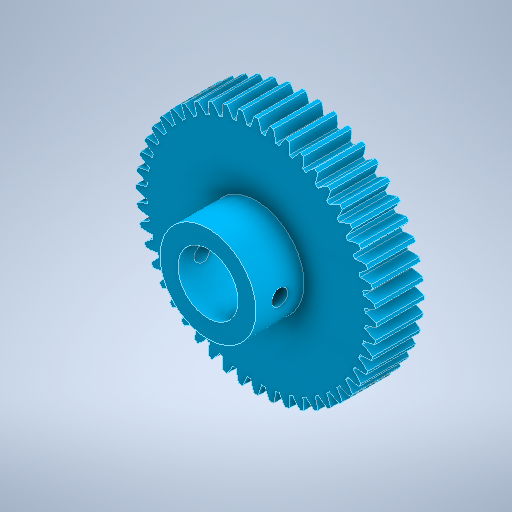
# Autodesk Inventor part: 平歯車2
Saved by Autodesk Inventor 2025.1 (Build 291241000, 241)
## iProperties
CustomPartVersion: 1
Created: 2024-10-03
Part Number: 平歯車2
Material: Steel
Document SubType Name: Modeling
Designer: yuki0520
Categories: <?xml version="1.0" encoding="UTF-16"?> <MemberInstance><Categories><FamilyTemplate><FamilyTemplateParameter ValueType="xs:double" Id="1" ObjectReferenceKey="da_z" ObjectType="kUserParameterObject"/><FamilyTemplateParameter ValueType="xs:double" Id="2" ObjectReferenceKey="da_b" ObjectType="kUserParameterObject"/><FamilyTemplateParameter ValueType="xs:double" Id="3" ObjectReferenceKey="da_beta" ObjectType="kUserParameterObject"/><FamilyTemplateParameter ValueType="xs:double" Id="4" ObjectReferenceKey="da_da" ObjectType="kUserParameterObject"/><FamilyTemplateParameter ValueType="xs:double" Id="5" ObjectReferenceKey="da_aw" ObjectType="kUserParameterObject"/><FamilyTemplateParameter ValueType="xs:string" Id="6" ObjectReferenceKey="EAIAABAAAACIAQAAAAAAAIAAAAAAAAAA" ObjectType="83910656" SubObjectId="SurfaceGeometry"/></FamilyTemplate><ParamToTemplateMap><ParamToTemplate CategoryParameter="//CategoryParameter[@InternalName='046C89C9-8512-4d59-83FE-43B91F4F132A']" TemplateParameter="1"/><ParamToTemplate CategoryParameter="//CategoryParameter[@InternalName='2552DF32-E462-4b46-AEBF-C6C7768E72AC']" TemplateParameter="2"/><ParamToTemplate CategoryParameter="//CategoryParameter[@InternalName='C9EE641D-15FC-4fae-A226-E94C4372FDD7']" TemplateParameter="3"/><ParamToTemplate><ParamToTemplate CategoryParameter="//CategoryParameter[@InternalName='00B6519A-459B-49c7-AD84-2E56D39A5744']" ConstantValue="0.000000"/></ParamToTemplate><ParamToTemplate><ParamToTemplate CategoryParameter="//CategoryParameter[@InternalName='04B31F0E-C7A6-4894-AA32-9629BEFACF47']" ConstantValue="1.000000"/></ParamToTemplate><ParamToTemplate><ParamToTemplate CategoryParameter="//CategoryParameter[@InternalName='43CBEC2E-7847-49e7-A936-2F7889FCB2D9']" ConstantValue="0.250000"/></ParamToTemplate><ParamToTemplate><ParamToTemplate CategoryParameter="//CategoryParameter[@InternalName='B1EFC894-105D-4ebd-86BF-FA20ED196853']" ConstantValue="0.350000"/></ParamToTemplate><ParamToTemplate><ParamToTemplate CategoryParameter="//CategoryParameter[@InternalName='51175063-3D10-4879-93E8-6246FE8B403D']" ConstantValue="2060000000.000000"/></ParamToTemplate><ParamToTemplate><ParamToTemplate CategoryParameter="//CategoryParameter[@InternalName='A3A52E27-4454-46a9-B0BD-C932399B70AF']" ConstantValue="0.300000"/></ParamToTemplate><ParamToTemplate><ParamToTemplate CategoryParameter="//CategoryParameter[@InternalName='91B76062-C214-41d9-B1B9-14D2AB99603D']" ConstantValue="0.100000"/></ParamToTemplate><ParamToTemplate><ParamToTemplate CategoryParameter="//CategoryParameter[@InternalName='374E806E-8B8A-4dda-A9AA-1039D6500AD2']" ConstantValue="10.000000"/></ParamToTemplate><ParamToTemplate><ParamToTemplate CategoryParameter="//CategoryParameter[@InternalName='2D373A89-B862-43d6-8D0B-0CBF12AB9F6C']" ConstantValue="0.349066"/></ParamToTemplate><ParamToTemplate CategoryParameter="//CategoryParameter[@InternalName='37777632-D6A2-4fac-9D53-DB8ACD95C989']" TemplateParameter="4"/><ParamToTemplate CategoryParameter="//CategoryParameter[@InternalName='FD1017F1-B727-4f7e-9707-0F86F1FF9423']" TemplateParameter="5"/><ParamToTemplate><ParamToTemplate CategoryParameter="//CategoryParameter[@InternalName='9E1B4470-B2D3-4ff1-B813-535BB4CDF51A']" ConstantValue="3520000.000000"/></ParamToTemplate><ParamToTemplate><ParamToTemplate CategoryParameter="//CategoryParameter[@InternalName='F8452263-BFF6-458c-9FB1-07C4B99E95CD']" ConstantValue="11400000.000000"/></ParamToTemplate><ParamToTemplate><ParamToTemplate CategoryParameter="//CategoryParameter[@InternalName='3E3BB259-FD49-497f-8171-6EBC954A3479']" ConstantValue="2.000000"/></ParamToTemplate><ParamToTemplate CategoryParameter="//CategoryParameter[@InternalName='27C3BAF2-7550-4e4b-AE2C-0DB134B7D9B7']" TemplateParameter="6"/></ParamToTemplateMap><Category DisplayName="Gear" InternalName="DC85795E-93AB-48d5-8EEE-5A27447B64BD" Mnemonic="Gear"><CategoryParameter DisplayName="z" InternalName="046C89C9-8512-4d59-83FE-43B91F4F132A" Mnemonic="z"/><CategoryParameter DisplayName="b" InternalName="2552DF32-E462-4b46-AEBF-C6C7768E72AC" Mnemonic="b"/><CategoryParameter DisplayName="||b|" InternalName="C9EE641D-15FC-4fae-A226-E94C4372FDD7" Mnemonic="beta"/><CategoryParameter DisplayName="x" InternalName="00B6519A-459B-49c7-AD84-2E56D39A5744" Mnemonic="x"/><CategoryParameter DisplayName="a*" InternalName="04B31F0E-C7A6-4894-AA32-9629BEFACF47" Mnemonic="a"/><CategoryParameter DisplayName="c*" InternalName="43CBEC2E-7847-49e7-A936-2F7889FCB2D9" Mnemonic="c"/><CategoryParameter DisplayName="r|.f|*" InternalName="B1EFC894-105D-4ebd-86BF-FA20ED196853" Mnemonic="rf"/><CategoryParameter DisplayName="E" InternalName="51175063-3D10-4879-93E8-6246FE8B403D" Mnemonic="E"/><CategoryParameter DisplayName="||m|" InternalName="A3A52E27-4454-46a9-B0BD-C932399B70AF" Mnemonic="mi"/><Category DisplayName="SpurGear" InternalName="26C5A22E-A91E-4dfd-A3B3-23CCAFAE1764" Mnemonic="SpurGear"><CategoryParameter DisplayName="m" InternalName="91B76062-C214-41d9-B1B9-14D2AB99603D" Mnemonic="m"/><CategoryParameter DisplayName="P" InternalName="374E806E-8B8A-4dda-A9AA-1039D6500AD2" Mnemonic="PP"/><CategoryParameter DisplayName="||a|" InternalName="2D373A89-B862-43d6-8D0B-0CBF12AB9F6C" Mnemonic="alpha"/><CategoryParameter DisplayName="d|.a|" InternalName="37777632-D6A2-4fac-9D53-DB8ACD95C989" Mnemonic="da"/><CategoryParameter DisplayName="a|.w|" InternalName="FD1017F1-B727-4f7e-9707-0F86F1FF9423" Mnemonic="aw"/><CategoryParameter DisplayName="||s||.Flim|" InternalName="9E1B4470-B2D3-4ff1-B813-535BB4CDF51A" Mnemonic="sFlim"/><CategoryParameter DisplayName="||s||.Hlim|" InternalName="F8452263-BFF6-458c-9FB1-07C4B99E95CD" Mnemonic="sHlim"/><CategoryParameter DisplayName="タイプ" InternalName="3E3BB259-FD49-497f-8171-6EBC954A3479" Mnemonic="type"/><CategoryParameter DisplayName="PitchDiameter" InternalName="27C3BAF2-7550-4e4b-AE2C-0DB134B7D9B7" Mnemonic="IDS_PITCHDIAM"/></Category></Category></Categories></MemberInstance>
Density: 1 g/cm^3
Appearance: スカイ ブルー 標準
Author: yuki0520
Autodesk Inventor part; units mm, degrees
sketch "Sketch1" plane through (0, 0, 0) normal (0, 0, 1) x (1, 0, 0)
  circle A0 centre (0, 0) radius 25
  dimension "d0" = 50
  constraints: 1 centre point
  measures "d0" diameter of A0
extrude "Extrusion1" add sketch "Sketch1" along normal blind 10
ref_plane "Work Plane2" through (0, 0, 5) normal (0, 0, 1) x (1, 0, 0)
sketch "Sketch2" plane through (0, 0, 0) normal (0, 0, -1) x (-1, 0, 0)
  circle A0 centre (0, 0) radius 25 projected
  circle A1 centre (0, 0) radius 24
  dimension "d3" = 48
  constraints: 1 centre point, 1 coincident
  measures "d3" diameter of A1
surface extrude "ピッチ円直径" sketch "Sketch2" against normal through all shown no curves A1
ref_plane "Work Plane8" through (0, 0, 0) normal (0.9978589, 0.0654031, 0) x (0, 0, 1)
ref_plane "Work Plane9" through (0, 0, 0) normal (1, 0, 0) x (0, 1, 0)
spur gear teeth "平歯車" teeth 48 pitch diameter 48 tip diameter 50 root diameter 45.5 face width 10 start plane through (0, 0, 0) normal (0, 0, -1) x (-1, 0, 0)
sketch "スケッチ3" plane through (0, 0, 10) normal (0, 0, 1) x (1, 0, 0)
  circle A0 centre (0, 0) radius 6
  circle A1 centre (0, 0) radius 10
  arc A2 (3.6683, -24.7294) -> (4.0726, -22.3825) centre (-7.7435, -21.5549) ccw projected
  arc A3 (4.0726, -22.3825) -> (4.8028, -22.2373) centre (0, 0) ccw projected
  arc A4 (4.8028, -22.2373) -> (6.0745, -24.2508) centre (15.4028, -16.9508) ccw projected
  arc A5 (6.0745, -24.2508) -> (6.8647, -24.039) centre (0, 0) ccw projected
  arc A6 (6.8647, -24.039) -> (6.9593, -21.6594) centre (-4.8638, -22.3812) ccw projected
  arc A7 (6.9593, -21.6594) -> (7.6642, -21.4201) centre (0, 0) ccw projected
  arc A8 (7.6642, -21.4201) -> (9.1879, -23.2504) centre (17.4835, -14.7953) ccw projected
  arc A9 (9.1879, -23.2504) -> (9.9437, -22.9374) centre (0, 0) ccw projected
  arc A10 (9.9437, -22.9374) -> (9.7269, -20.5658) centre (-1.9009, -22.8246) ccw projected
  arc A11 (9.7269, -20.5658) -> (10.3946, -20.2365) centre (0, 0) ccw projected
  arc A12 (10.3946, -20.2365) -> (12.1441, -21.8523) centre (19.2651, -12.3867) ccw projected
  arc A13 (12.1441, -21.8523) -> (12.8526, -21.4432) centre (0, 0) ccw projected
  arc A14 (12.8526, -21.4432) -> (12.328, -19.1202) centre (1.0946, -22.8774) ccw projected
  arc A15 (12.328, -19.1202) -> (12.947, -18.7066) centre (0, 0) ccw projected
  arc A16 (12.947, -18.7066) -> (14.8925, -20.0802) centre (20.7171, -9.7661) ccw projected
  arc A17 (14.8925, -20.0802) -> (15.5415, -19.5822) centre (0, 0) ccw projected
  arc A18 (15.5415, -19.5822) -> (14.7183, -17.3475) centre (4.0714, -22.5388) ccw projected
  arc A19 (14.7183, -17.3475) -> (15.278, -16.8566) centre (0, 0) ccw projected
  arc A20 (15.278, -16.8566) -> (17.3861, -17.9645) centre (21.8146, -6.9784) ccw projected
  arc A21 (17.3861, -17.9645) -> (17.9645, -17.3861) centre (0, 0) ccw projected
  arc A22 (17.9645, -17.3861) -> (16.8566, -15.278) centre (6.9784, -21.8146) ccw projected
  arc A23 (16.8566, -15.278) -> (17.3475, -14.7183) centre (0, 0) ccw projected
  arc A24 (17.3475, -14.7183) -> (19.5822, -15.5415) centre (22.5388, -4.0714) ccw projected
  arc A25 (19.5822, -15.5415) -> (20.0802, -14.8925) centre (0, 0) ccw projected
  arc A26 (20.0802, -14.8925) -> (18.7066, -12.947) centre (9.7661, -20.7171) ccw projected
  arc A27 (18.7066, -12.947) -> (19.1202, -12.328) centre (0, 0) ccw projected
  arc A28 (19.1202, -12.328) -> (21.4432, -12.8526) centre (22.8774, -1.0946) ccw projected
  arc A29 (21.4432, -12.8526) -> (21.8523, -12.1441) centre (0, 0) ccw projected
  arc A30 (21.8523, -12.1441) -> (20.2365, -10.3946) centre (12.3867, -19.2651) ccw projected
  arc A31 (20.2365, -10.3946) -> (20.5658, -9.7269) centre (0, 0) ccw projected
  arc A32 (20.5658, -9.7269) -> (22.9374, -9.9437) centre (22.8246, 1.9009) ccw projected
  arc A33 (22.9374, -9.9437) -> (23.2504, -9.1879) centre (0, 0) ccw projected
  arc A34 (23.2504, -9.1879) -> (21.4201, -7.6642) centre (14.7953, -17.4835) ccw projected
  arc A35 (21.4201, -7.6642) -> (21.6594, -6.9593) centre (0, 0) ccw projected
  arc A36 (21.6594, -6.9593) -> (24.039, -6.8647) centre (22.3812, 4.8638) ccw projected
  arc A37 (24.039, -6.8647) -> (24.2508, -6.0745) centre (0, 0) ccw projected
  arc A38 (24.2508, -6.0745) -> (22.2373, -4.8028) centre (16.9508, -15.4028) ccw projected
  arc A39 (22.2373, -4.8028) -> (22.3825, -4.0726) centre (0, 0) ccw projected
  arc A40 (22.3825, -4.0726) -> (24.7294, -3.6683) centre (21.5549, 7.7435) ccw projected
  arc A41 (24.7294, -3.6683) -> (24.8362, -2.8572) centre (0, 0) ccw projected
  arc A42 (24.8362, -2.8572) -> (22.6739, -1.8592) centre (18.8162, -13.0585) ccw projected
  arc A43 (22.6739, -1.8592) -> (22.7226, -1.1163) centre (0, 0) ccw projected
  arc A44 (22.7226, -1.1163) -> (24.9967, -0.409) centre (20.3597, 10.4907) ccw projected
  arc A45 (24.9967, -0.409) -> (24.9967, 0.409) centre (0, 0) ccw projected
  arc A46 (24.9967, 0.409) -> (22.7226, 1.1163) centre (20.3597, -10.4907) ccw projected
  arc A47 (22.7226, 1.1163) -> (22.6739, 1.8592) centre (0, 0) ccw projected
  arc A48 (22.6739, 1.8592) -> (24.8362, 2.8572) centre (18.8162, 13.0585) ccw projected
  arc A49 (24.8362, 2.8572) -> (24.7294, 3.6683) centre (0, 0) ccw projected
  arc A50 (24.7294, 3.6683) -> (22.3825, 4.0726) centre (21.5549, -7.7435) ccw projected
  arc A51 (22.3825, 4.0726) -> (22.2373, 4.8028) centre (0, 0) ccw projected
  arc A52 (22.2373, 4.8028) -> (24.2508, 6.0745) centre (16.9508, 15.4028) ccw projected
  arc A53 (24.2508, 6.0745) -> (24.039, 6.8647) centre (0, 0) ccw projected
  arc A54 (24.039, 6.8647) -> (21.6594, 6.9593) centre (22.3812, -4.8638) ccw projected
  arc A55 (21.6594, 6.9593) -> (21.4201, 7.6642) centre (0, 0) ccw projected
  arc A56 (21.4201, 7.6642) -> (23.2504, 9.1879) centre (14.7953, 17.4835) ccw projected
  arc A57 (23.2504, 9.1879) -> (22.9374, 9.9437) centre (0, 0) ccw projected
  arc A58 (22.9374, 9.9437) -> (20.5658, 9.7269) centre (22.8246, -1.9009) ccw projected
  arc A59 (20.5658, 9.7269) -> (20.2365, 10.3946) centre (0, 0) ccw projected
  arc A60 (20.2365, 10.3946) -> (21.8523, 12.1441) centre (12.3867, 19.2651) ccw projected
  arc A61 (21.8523, 12.1441) -> (21.4432, 12.8526) centre (0, 0) ccw projected
  arc A62 (21.4432, 12.8526) -> (19.1202, 12.328) centre (22.8774, 1.0946) ccw projected
  arc A63 (19.1202, 12.328) -> (18.7066, 12.947) centre (0, 0) ccw projected
  arc A64 (18.7066, 12.947) -> (20.0802, 14.8925) centre (9.7661, 20.7171) ccw projected
  arc A65 (20.0802, 14.8925) -> (19.5822, 15.5415) centre (0, 0) ccw projected
  arc A66 (19.5822, 15.5415) -> (17.3475, 14.7183) centre (22.5388, 4.0714) ccw projected
  arc A67 (17.3475, 14.7183) -> (16.8566, 15.278) centre (0, 0) ccw projected
  arc A68 (16.8566, 15.278) -> (17.9645, 17.3861) centre (6.9784, 21.8146) ccw projected
  arc A69 (17.9645, 17.3861) -> (17.3861, 17.9645) centre (0, 0) ccw projected
  arc A70 (17.3861, 17.9645) -> (15.278, 16.8566) centre (21.8146, 6.9784) ccw projected
  arc A71 (15.278, 16.8566) -> (14.7183, 17.3475) centre (0, 0) ccw projected
  arc A72 (14.7183, 17.3475) -> (15.5415, 19.5822) centre (4.0714, 22.5388) ccw projected
  arc A73 (15.5415, 19.5822) -> (14.8925, 20.0802) centre (0, 0) ccw projected
  arc A74 (14.8925, 20.0802) -> (12.947, 18.7066) centre (20.7171, 9.7661) ccw projected
  arc A75 (12.947, 18.7066) -> (12.328, 19.1202) centre (0, 0) ccw projected
  arc A76 (12.328, 19.1202) -> (12.8526, 21.4432) centre (1.0946, 22.8774) ccw projected
  arc A77 (12.8526, 21.4432) -> (12.1441, 21.8523) centre (0, 0) ccw projected
  arc A78 (12.1441, 21.8523) -> (10.3946, 20.2365) centre (19.2651, 12.3867) ccw projected
  arc A79 (10.3946, 20.2365) -> (9.7269, 20.5658) centre (0, 0) ccw projected
  arc A80 (9.7269, 20.5658) -> (9.9437, 22.9374) centre (-1.9009, 22.8246) ccw projected
  arc A81 (9.9437, 22.9374) -> (9.1879, 23.2504) centre (0, 0) ccw projected
  arc A82 (9.1879, 23.2504) -> (7.6642, 21.4201) centre (17.4835, 14.7953) ccw projected
  arc A83 (7.6642, 21.4201) -> (6.9593, 21.6594) centre (0, 0) ccw projected
  arc A84 (6.9593, 21.6594) -> (6.8647, 24.039) centre (-4.8638, 22.3812) ccw projected
  arc A85 (6.8647, 24.039) -> (6.0745, 24.2508) centre (0, 0) ccw projected
  arc A86 (6.0745, 24.2508) -> (4.8028, 22.2373) centre (15.4028, 16.9508) ccw projected
  arc A87 (4.8028, 22.2373) -> (4.0726, 22.3825) centre (0, 0) ccw projected
  arc A88 (4.0726, 22.3825) -> (3.6683, 24.7294) centre (-7.7435, 21.5549) ccw projected
  arc A89 (3.6683, 24.7294) -> (2.8572, 24.8362) centre (0, 0) ccw projected
  arc A90 (2.8572, 24.8362) -> (1.8592, 22.6739) centre (13.0585, 18.8162) ccw projected
  arc A91 (1.8592, 22.6739) -> (1.1163, 22.7226) centre (0, 0) ccw projected
  arc A92 (1.1163, 22.7226) -> (0.409, 24.9967) centre (-10.4907, 20.3597) ccw projected
  arc A93 (0.409, 24.9967) -> (-0.409, 24.9967) centre (0, 0) ccw projected
  arc A94 (-0.409, 24.9967) -> (-1.1163, 22.7226) centre (10.4907, 20.3597) ccw projected
  arc A95 (-1.1163, 22.7226) -> (-1.8592, 22.6739) centre (0, 0) ccw projected
  arc A96 (-1.8592, 22.6739) -> (-2.8572, 24.8362) centre (-13.0585, 18.8162) ccw projected
  arc A97 (2.8572, -24.8362) -> (3.6683, -24.7294) centre (0, 0) ccw projected
  arc A98 (-3.6683, 24.7294) -> (-4.0726, 22.3825) centre (7.7435, 21.5549) ccw projected
  arc A99 (-4.0726, 22.3825) -> (-4.8028, 22.2373) centre (0, 0) ccw projected
  arc A100 (-4.8028, 22.2373) -> (-6.0745, 24.2508) centre (-15.4028, 16.9508) ccw projected
  arc A101 (-6.0745, 24.2508) -> (-6.8647, 24.039) centre (0, 0) ccw projected
  arc A102 (-6.8647, 24.039) -> (-6.9593, 21.6594) centre (4.8638, 22.3812) ccw projected
  arc A103 (-6.9593, 21.6594) -> (-7.6642, 21.4201) centre (0, 0) ccw projected
  arc A104 (-7.6642, 21.4201) -> (-9.1879, 23.2504) centre (-17.4835, 14.7953) ccw projected
  arc A105 (-9.1879, 23.2504) -> (-9.9437, 22.9374) centre (0, 0) ccw projected
  arc A106 (-9.9437, 22.9374) -> (-9.7269, 20.5658) centre (1.9009, 22.8246) ccw projected
  arc A107 (-9.7269, 20.5658) -> (-10.3946, 20.2365) centre (0, 0) ccw projected
  arc A108 (-10.3946, 20.2365) -> (-12.1441, 21.8523) centre (-19.2651, 12.3867) ccw projected
  arc A109 (-12.1441, 21.8523) -> (-12.8526, 21.4432) centre (0, 0) ccw projected
  arc A110 (-12.8526, 21.4432) -> (-12.328, 19.1202) centre (-1.0946, 22.8774) ccw projected
  arc A111 (-12.328, 19.1202) -> (-12.947, 18.7066) centre (0, 0) ccw projected
  arc A112 (-12.947, 18.7066) -> (-14.8925, 20.0802) centre (-20.7171, 9.7661) ccw projected
  arc A113 (-14.8925, 20.0802) -> (-15.5415, 19.5822) centre (0, 0) ccw projected
  arc A114 (-15.5415, 19.5822) -> (-14.7183, 17.3475) centre (-4.0714, 22.5388) ccw projected
  arc A115 (-14.7183, 17.3475) -> (-15.278, 16.8566) centre (0, 0) ccw projected
  arc A116 (-15.278, 16.8566) -> (-17.3861, 17.9645) centre (-21.8146, 6.9784) ccw projected
  arc A117 (-17.3861, 17.9645) -> (-17.9645, 17.3861) centre (0, 0) ccw projected
  arc A118 (-17.9645, 17.3861) -> (-16.8566, 15.278) centre (-6.9784, 21.8146) ccw projected
  arc A119 (-16.8566, 15.278) -> (-17.3475, 14.7183) centre (0, 0) ccw projected
  arc A120 (-17.3475, 14.7183) -> (-19.5822, 15.5415) centre (-22.5388, 4.0714) ccw projected
  arc A121 (-19.5822, 15.5415) -> (-20.0802, 14.8925) centre (0, 0) ccw projected
  arc A122 (-20.0802, 14.8925) -> (-18.7066, 12.947) centre (-9.7661, 20.7171) ccw projected
  arc A123 (-18.7066, 12.947) -> (-19.1202, 12.328) centre (0, 0) ccw projected
  arc A124 (-19.1202, 12.328) -> (-21.4432, 12.8526) centre (-22.8774, 1.0946) ccw projected
  arc A125 (-21.4432, 12.8526) -> (-21.8523, 12.1441) centre (0, 0) ccw projected
  arc A126 (-21.8523, 12.1441) -> (-20.2365, 10.3946) centre (-12.3867, 19.2651) ccw projected
  arc A127 (-20.2365, 10.3946) -> (-20.5658, 9.7269) centre (0, 0) ccw projected
  arc A128 (-20.5658, 9.7269) -> (-22.9374, 9.9437) centre (-22.8246, -1.9009) ccw projected
  arc A129 (-22.9374, 9.9437) -> (-23.2504, 9.1879) centre (0, 0) ccw projected
  arc A130 (-23.2504, 9.1879) -> (-21.4201, 7.6642) centre (-14.7953, 17.4835) ccw projected
  arc A131 (-21.4201, 7.6642) -> (-21.6594, 6.9593) centre (0, 0) ccw projected
  arc A132 (-21.6594, 6.9593) -> (-24.039, 6.8647) centre (-22.3812, -4.8638) ccw projected
  arc A133 (-24.039, 6.8647) -> (-24.2508, 6.0745) centre (0, 0) ccw projected
  arc A134 (-24.2508, 6.0745) -> (-22.2373, 4.8028) centre (-16.9508, 15.4028) ccw projected
  arc A135 (-22.2373, 4.8028) -> (-22.3825, 4.0726) centre (0, 0) ccw projected
  arc A136 (-22.3825, 4.0726) -> (-24.7294, 3.6683) centre (-21.5549, -7.7435) ccw projected
  arc A137 (-24.7294, 3.6683) -> (-24.8362, 2.8572) centre (0, 0) ccw projected
  arc A138 (-24.8362, 2.8572) -> (-22.6739, 1.8592) centre (-18.8162, 13.0585) ccw projected
  arc A139 (-22.6739, 1.8592) -> (-22.7226, 1.1163) centre (0, 0) ccw projected
  arc A140 (-22.7226, 1.1163) -> (-24.9967, 0.409) centre (-20.3597, -10.4907) ccw projected
  arc A141 (-24.9967, 0.409) -> (-24.9967, -0.409) centre (0, 0) ccw projected
  arc A142 (-24.9967, -0.409) -> (-22.7226, -1.1163) centre (-20.3597, 10.4907) ccw projected
  arc A143 (-22.7226, -1.1163) -> (-22.6739, -1.8592) centre (0, 0) ccw projected
  arc A144 (-22.6739, -1.8592) -> (-24.8362, -2.8572) centre (-18.8162, -13.0585) ccw projected
  arc A145 (-24.8362, -2.8572) -> (-24.7294, -3.6683) centre (0, 0) ccw projected
  arc A146 (-24.7294, -3.6683) -> (-22.3825, -4.0726) centre (-21.5549, 7.7435) ccw projected
  arc A147 (-22.3825, -4.0726) -> (-22.2373, -4.8028) centre (0, 0) ccw projected
  arc A148 (-22.2373, -4.8028) -> (-24.2508, -6.0745) centre (-16.9508, -15.4028) ccw projected
  arc A149 (-24.2508, -6.0745) -> (-24.039, -6.8647) centre (0, 0) ccw projected
  arc A150 (-24.039, -6.8647) -> (-21.6594, -6.9593) centre (-22.3812, 4.8638) ccw projected
  arc A151 (-21.6594, -6.9593) -> (-21.4201, -7.6642) centre (0, 0) ccw projected
  arc A152 (-21.4201, -7.6642) -> (-23.2504, -9.1879) centre (-14.7953, -17.4835) ccw projected
  arc A153 (-23.2504, -9.1879) -> (-22.9374, -9.9437) centre (0, 0) ccw projected
  arc A154 (-22.9374, -9.9437) -> (-20.5658, -9.7269) centre (-22.8246, 1.9009) ccw projected
  arc A155 (-20.5658, -9.7269) -> (-20.2365, -10.3946) centre (0, 0) ccw projected
  arc A156 (-20.2365, -10.3946) -> (-21.8523, -12.1441) centre (-12.3867, -19.2651) ccw projected
  arc A157 (-21.8523, -12.1441) -> (-21.4432, -12.8526) centre (0, 0) ccw projected
  arc A158 (-21.4432, -12.8526) -> (-19.1202, -12.328) centre (-22.8774, -1.0946) ccw projected
  arc A159 (-19.1202, -12.328) -> (-18.7066, -12.947) centre (0, 0) ccw projected
  arc A160 (-18.7066, -12.947) -> (-20.0802, -14.8925) centre (-9.7661, -20.7171) ccw projected
  arc A161 (-20.0802, -14.8925) -> (-19.5822, -15.5415) centre (0, 0) ccw projected
  arc A162 (-19.5822, -15.5415) -> (-17.3475, -14.7183) centre (-22.5388, -4.0714) ccw projected
  arc A163 (-17.3475, -14.7183) -> (-16.8566, -15.278) centre (0, 0) ccw projected
  arc A164 (-16.8566, -15.278) -> (-17.9645, -17.3861) centre (-6.9784, -21.8146) ccw projected
  arc A165 (-17.9645, -17.3861) -> (-17.3861, -17.9645) centre (0, 0) ccw projected
  arc A166 (-17.3861, -17.9645) -> (-15.278, -16.8566) centre (-21.8146, -6.9784) ccw projected
  arc A167 (-15.278, -16.8566) -> (-14.7183, -17.3475) centre (0, 0) ccw projected
  arc A168 (-14.7183, -17.3475) -> (-15.5415, -19.5822) centre (-4.0714, -22.5388) ccw projected
  arc A169 (-15.5415, -19.5822) -> (-14.8925, -20.0802) centre (0, 0) ccw projected
  arc A170 (-14.8925, -20.0802) -> (-12.947, -18.7066) centre (-20.7171, -9.7661) ccw projected
  arc A171 (-12.947, -18.7066) -> (-12.328, -19.1202) centre (0, 0) ccw projected
  arc A172 (-12.328, -19.1202) -> (-12.8526, -21.4432) centre (-1.0946, -22.8774) ccw projected
  arc A173 (-12.8526, -21.4432) -> (-12.1441, -21.8523) centre (0, 0) ccw projected
  arc A174 (-12.1441, -21.8523) -> (-10.3946, -20.2365) centre (-19.2651, -12.3867) ccw projected
  arc A175 (-10.3946, -20.2365) -> (-9.7269, -20.5658) centre (0, 0) ccw projected
  arc A176 (-9.7269, -20.5658) -> (-9.9437, -22.9374) centre (1.9009, -22.8246) ccw projected
  arc A177 (-9.9437, -22.9374) -> (-9.1879, -23.2504) centre (0, 0) ccw projected
  arc A178 (-9.1879, -23.2504) -> (-7.6642, -21.4201) centre (-17.4835, -14.7953) ccw projected
  arc A179 (-7.6642, -21.4201) -> (-6.9593, -21.6594) centre (0, 0) ccw projected
  arc A180 (-6.9593, -21.6594) -> (-6.8647, -24.039) centre (4.8638, -22.3812) ccw projected
  arc A181 (-6.8647, -24.039) -> (-6.0745, -24.2508) centre (0, 0) ccw projected
  arc A182 (-6.0745, -24.2508) -> (-4.8028, -22.2373) centre (-15.4028, -16.9508) ccw projected
  arc A183 (-4.8028, -22.2373) -> (-4.0726, -22.3825) centre (0, 0) ccw projected
  arc A184 (-4.0726, -22.3825) -> (-3.6683, -24.7294) centre (7.7435, -21.5549) ccw projected
  arc A185 (-3.6683, -24.7294) -> (-2.8572, -24.8362) centre (0, 0) ccw projected
  arc A186 (-2.8572, -24.8362) -> (-1.8592, -22.6739) centre (-13.0585, -18.8162) ccw projected
  arc A187 (-1.8592, -22.6739) -> (-1.1163, -22.7226) centre (0, 0) ccw projected
  arc A188 (-1.1163, -22.7226) -> (-0.409, -24.9967) centre (10.4907, -20.3597) ccw projected
  arc A189 (-0.409, -24.9967) -> (0.409, -24.9967) centre (0, 0) ccw projected
  arc A190 (0.409, -24.9967) -> (1.1163, -22.7226) centre (-10.4907, -20.3597) ccw projected
  arc A191 (1.1163, -22.7226) -> (1.8592, -22.6739) centre (0, 0) ccw projected
  arc A192 (1.8592, -22.6739) -> (2.8572, -24.8362) centre (13.0585, -18.8162) ccw projected
  arc A193 (-2.8572, 24.8362) -> (-3.6683, 24.7294) centre (0, 0) ccw projected
  dimension "d49" = 12
  dimension "d50" = 4
  constraints: 2 centre point, 1 coincident
  measures "d49" diameter of A0
  measures "d50" radial gap between concentric circles of A0 A1
extrude "押し出し2" add sketch "スケッチ3" along normal blind 10 contours A0 | A1
sketch "スケッチ4" plane through (0, 0, 0) normal (0, 0, -1) x (-1, 0, 0)
  circle A0 centre (0, 0) radius 6.25
  dimension "d53" = 12.5
  constraints: 1 centre point, 1 coincident
  measures "d53" diameter of A0
extrude "押し出し3" cut sketch "スケッチ4" against normal blind 100
sketch "スケッチ5" plane through (0, 0, 0) normal (1, 0, 0) x (0, 1, 0)
  line L0 (22.6739, 0) -> (22.7226, 0) projected
  line L1 (22.7226, 0) -> (22.7226, 10) projected
  line L2 (-6.25, 20) -> (6.25, 20) projected
  line L3 (22.7226, 10) -> (22.6739, 10) projected
  line L4 (22.6739, 0) -> (22.6739, 10) projected
  line L5 (10, 20) -> (-10, 20) projected
  line L6 (-10, 10) -> (10, 10) projected
  line L7 (0, 20) -> (0, 10)
  point P0 (0, 0)
  point P1 (22.75, 20)
  point P2 (-22.75, 20)
  point P3 (0, 15)
  dimension "d65" = 5
  dimension "d66" = 10
  constraints: 3 midpoint, 2 end point
  measures "d65" distance from line of point (0, 15) L2
  measures "d66" distance of L7.start L7.end
hole "穴1" at (0, 0, 15) direction (-1, 0, 0) diameter 3.3 end through all both
equation "\"d0\" = da_da"
equation "\"d1\" = da_b"
equation "\"d3\" = da_d"
equation "\"d16\" = da_aw"
equation "\"d43\" = da_aw"
equation "\"d46\" = da_aw"
equation "\"da_da\" = 50"
equation "\"da_b\" = 10"
equation "\"da_d\" = 48"
equation "\"da_aw\" = 48"
body "Solid1"
body "Srf1"
